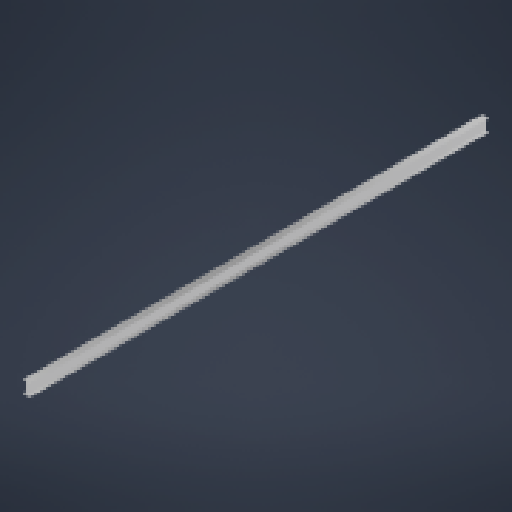
# Autodesk Inventor part: Floor Frame, I Section
Saved by Autodesk Inventor 2026 (Build 300175000, 175)
## iProperties
Created: 2025-11-04
Part Number: Floor Frame, I Section
Material: Aluminum 6061
Document SubType Name: Modeling
Designer: Brandon Portillo
Density: 2.7 g/cm^3
Appearance: Aluminum - Flat
Author: Brandon Portillo
Autodesk Inventor part; units mm, degrees
ref_plane "YZ Plane" through (0, 0, 0) normal (1, 0, 0) x (0, 1, 0)
ref_plane "XZ Plane" through (0, 0, 0) normal (0, 1, 0) x (-1, 0, 0)
ref_plane "XY Plane" through (0, 0, 0) normal (0, 0, 1) x (1, 0, 0)
sketch "Sketch1" plane through (0, 0, 0) normal (0, 0, 1) x (1, 0, 0)
  line L0 (0, 0) -> (4, 0)
  line L1 (4, 0) -> (4, 90)
  line L2 (4, 90) -> (0, 90)
  line L3 (0, 90) -> (0, 0)
  line L4 (-23, 92.5) -> (27, 92.5)
  line L5 (27, 92.5) -> (27, 87.5)
  line L6 (27, 87.5) -> (-23, 87.5)
  line L7 (-23, 87.5) -> (-23, 92.5)
  line L8 (-23, 92.5) -> (27, 87.5) construction
  line L9 (27, 92.5) -> (-23, 87.5) construction
  line L10 (-23, -2.5) -> (27, -2.5)
  line L11 (27, -2.5) -> (27, 2.5)
  line L12 (27, 2.5) -> (-23, 2.5)
  line L13 (-23, 2.5) -> (-23, -2.5)
  line L14 (-23, -2.5) -> (27, 2.5) construction
  line L15 (27, -2.5) -> (-23, 2.5) construction
  point P0 (2, 90)
  point P1 (2, 0)
  point P2 (4, 87.5)
  point P3 (0, 87.5)
  point P4 (0, 2.5)
  point P5 (4, 2.5)
  dimension "d0" = 4
  dimension "d1" = 90
  dimension "d2" = 50
  dimension "d3" = 5
  dimension "d4" = 50
  dimension "d5" = 5
  constraints: 32 end point, 6 midpoint, 6 parallel, 3 horizontal, 3 perpendicular
  measures "d0" distance of L2.end L1.end
  measures "d1" distance of L1.end L0.end
  measures "d2" distance of L5.end L6.end
  measures "d3" distance of L4.end L5.end
  measures "d4" distance of L12.end L11.end
  measures "d5" distance of L11.end L10.end
extrude "Extrusion1" add sketch "Sketch1" along normal blind 3730
body "Solid1"
